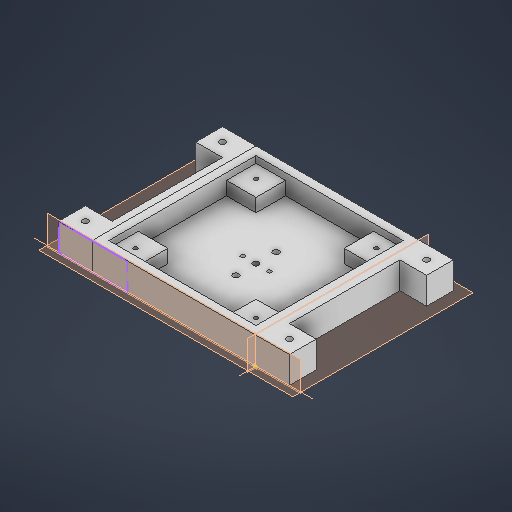
# Autodesk Inventor part: Unterteil
Saved by Autodesk Inventor 2026.2 (Build 302298000, 298)
## iProperties
Created: 2026-04-09
Part Number: Unterteil
Material: Generisch
Document SubType Name: Modeling
Designer: linda
Density: 1 g/cm^3
Appearance: Vorgabe
Author: linda
Autodesk Inventor part; units mm, degrees
sketch "Skizze1" plane through (0, 0, 0) normal (0, 1, 0) x (-1, 0, 0)
  line L0 (0, 0) -> (122.5, 0)
  line L1 (122.5, 0) -> (122.5, -122.5)
  line L2 (122.5, -122.5) -> (0, -122.5)
  line L3 (0, -122.5) -> (0, 0)
  dimension "d0" = 122.5
  dimension "d1" = 122.5
  constraints: 8 end point, 2 parallel, 1 horizontal, 1 perpendicular
  measures "d0" distance of L1.end L2.end
  measures "d1" distance of L0.end L1.end
extrude "Extrusion1" add sketch "Skizze1" along normal blind 20
sketch "Skizze2" plane through (0, 20, 0) normal (0, 1, 0) x (1, 0, 0)
  line L0 (-6.25042, 6.249757) -> (-116.25042, 6.249757)
  line L1 (-116.25042, 6.249757) -> (-116.25042, 116.249757)
  line L2 (-116.25042, 116.249757) -> (-6.25042, 116.249757)
  line L3 (-6.25042, 116.249757) -> (-6.25042, 6.249757)
  point P0 (0, 0)
  dimension "d6" = 110
  dimension "d7" = 110
  constraints: 8 end point, 2 parallel, 1 horizontal, 1 perpendicular
  measures "d6" distance of L1.end L2.end
  measures "d7" distance of L0.end L1.end
extrude "Extrusion2" cut sketch "Skizze2" against normal blind 15
sketch "Skizze3" plane through (0, 5, 0) normal (0, 1, 0) x (1, 0, 0)
  line L0 (-6.250425, 6.249784) -> (-21.250425, 6.249784)
  line L1 (-21.250425, 6.249784) -> (-21.250425, 21.249784)
  line L2 (-21.250425, 21.249784) -> (-6.250425, 21.249784)
  line L3 (-6.250425, 21.249784) -> (-6.250425, 6.249784)
  line L4 (-6.250425, 116.250797) -> (-21.250425, 116.250797)
  line L5 (-21.250425, 116.250797) -> (-21.250425, 101.250797)
  line L6 (-21.250425, 101.250797) -> (-6.250425, 101.250797)
  line L7 (-6.250425, 101.250797) -> (-6.250425, 116.250797)
  line L8 (-116.250374, 116.249733) -> (-101.250374, 116.249733)
  line L9 (-101.250374, 116.249733) -> (-101.250374, 101.249733)
  line L10 (-101.250374, 101.249733) -> (-116.250374, 101.249733)
  line L11 (-116.250374, 101.249733) -> (-116.250374, 116.249733)
  line L12 (-116.250374, 6.249784) -> (-101.250374, 6.249784)
  line L13 (-101.250374, 6.249784) -> (-101.250374, 21.249784)
  line L14 (-101.250374, 21.249784) -> (-116.250374, 21.249784)
  line L15 (-116.250374, 21.249784) -> (-116.250374, 6.249784)
  point P0 (0, 0)
  dimension "d10" = 15
  dimension "d11" = 15
  dimension "d12" = 15
  dimension "d13" = 15
  dimension "d14" = 15
  dimension "d15" = 15
  dimension "d16" = 15
  dimension "d17" = 15
  constraints: 32 end point, 8 parallel, 4 horizontal, 4 perpendicular, 1 point on line
  measures "d10" distance of L1.end L2.end
  measures "d11" distance of L0.end L1.end
  measures "d12" distance of L6.end L5.end
  measures "d13" distance of L5.end L4.end
  measures "d14" distance of L9.end L10.end
  measures "d15" distance of L8.end L9.end
  measures "d16" distance of L14.end L13.end
  measures "d17" distance of L13.end L12.end
extrude "Extrusion3" add sketch "Skizze3" along normal blind 10
sketch "Skizze4" plane through (0, 5, 0) normal (0, 1, 0) x (1, 0, 0)
  line L0 (-21.249763, 21.249862) -> (-28.320831, 28.32093)
  line L1 (-21.249763, 21.249862) -> (-11.249763, 21.249862) construction
  line L2 (-28.320831, 28.32093) -> (-6.25074, 28.32093)
  line L3 (-6.25074, 28.32093) -> (-6.25074, 6.250839)
  line L4 (-6.25074, 6.250839) -> (-28.320831, 6.250839)
  line L5 (-28.320831, 6.250839) -> (-28.320831, 28.32093)
  line L6 (-21.250382, 101.250909) -> (-28.32145, 94.179842)
  line L7 (-21.250382, 101.250909) -> (-11.250382, 101.250909) construction
  line L8 (-6.250411, 116.249742) -> (-28.32145, 116.249742)
  line L9 (-28.32145, 116.249742) -> (-28.32145, 94.179842)
  line L10 (-28.32145, 94.179842) -> (-6.250411, 94.179842)
  line L11 (-6.250411, 94.179842) -> (-6.250411, 116.249742)
  line L12 (-101.251429, 21.249862) -> (-94.180362, 28.32093)
  line L13 (-101.251429, 21.249862) -> (-91.251429, 21.249862) construction
  line L14 (-94.180362, 28.32093) -> (-116.250453, 28.32093)
  line L15 (-116.250453, 28.32093) -> (-116.250453, 6.250839)
  line L16 (-116.250453, 6.250839) -> (-94.180362, 6.250839)
  line L17 (-94.180362, 6.250839) -> (-94.180362, 28.32093)
  line L18 (-101.251429, 101.250909) -> (-94.180362, 94.179842)
  line L19 (-101.251429, 101.250909) -> (-91.251429, 101.250909) construction
  line L20 (-94.180362, 94.179842) -> (-116.250453, 94.179842)
  line L21 (-116.250453, 94.179842) -> (-116.250453, 116.249933)
  line L22 (-116.250453, 116.249933) -> (-94.180362, 116.249933)
  line L23 (-94.180362, 116.249933) -> (-94.180362, 94.179842)
  point P0 (0, 0)
  dimension "d20" = 10
  dimension "d21" = 135
  dimension "d22" = 10
  dimension "d23" = 135
  dimension "d24" = 10
  dimension "d25" = 45
  dimension "d26" = 10
  dimension "d27" = 45
  constraints: 48 end point, 8 horizontal, 8 parallel, 4 equal length, 4 perpendicular, 2 point on line
  measures "d20" distance of L0.start L0.end
  measures "d21" angle of L1 L0
  measures "d22" distance of L6.start L6.end
  measures "d23" angle of L6 L7
  measures "d24" distance of L12.start L12.end
  measures "d25" angle of L13 L12
  measures "d26" distance of L18.start L18.end
  measures "d27" angle of L18 L19
extrude "Extrusion4" add sketch "Skizze4" along normal blind 10
sketch "Skizze5" plane through (0, 15, 0) normal (0, 1, 0) x (1, 0, 0)
  line L0 (-28.320831, 28.32093) -> (-28.320831, 6.250839)
  line L1 (-6.25074, 28.32093) -> (-28.320831, 28.32093)
  point P0 (0, 0)
  point P1 (-16.250831, 16.25093)
  dimension "d30" = 12.07
  dimension "d31" = 12.07
  measures "d30" distance from line of L0 point (-16.251, 16.251)
  measures "d31" distance from line of L1 point (-16.251, 16.251)
hole "Bohrung1" at (-16.250831, 15, -16.25093) direction (0, -1, 0) diameter 3 end through all
sketch "Skizze6" plane through (0, 15, 0) normal (0, 1, 0) x (1, 0, 0)
  line L0 (-94.180362, 6.250839) -> (-94.180362, 28.32093)
  line L1 (-94.180362, 28.32093) -> (-116.25042, 28.32093)
  point P0 (0, 0)
  point P1 (-106.250362, 16.25093)
  dimension "d39" = 12.07
  dimension "d40" = 12.07
  measures "d39" distance from line of L0 point (-106.25, 16.251)
  measures "d40" distance from line of L1 point (-106.25, 16.251)
hole "Bohrung2" at (-106.250362, 15, -16.25093) direction (0, -1, 0) diameter 3 end through all
sketch "Skizze7" plane through (0, 15, 0) normal (0, 1, 0) x (1, 0, 0)
  line L0 (-28.32145, 94.179842) -> (-6.25042, 94.179842)
  line L1 (-28.32145, 116.249742) -> (-28.32145, 94.179842)
  point P0 (0, 0)
  point P1 (-16.25145, 106.249842)
  dimension "d48" = 12.07
  dimension "d49" = 12.07
  measures "d48" distance from line of L0 point (-16.251, 106.25)
  measures "d49" distance from line of L1 point (-16.251, 106.25)
hole "Bohrung3" at (-16.25145, 15, -106.249842) direction (0, -1, 0) diameter 3 end through all
sketch "Skizze8" plane through (0, 15, 0) normal (0, 1, 0) x (1, 0, 0)
  line L0 (-116.25042, 94.179842) -> (-94.180362, 94.179842)
  line L1 (-94.180362, 94.179842) -> (-94.180362, 116.249757)
  point P0 (0, 0)
  point P1 (-106.250362, 106.249842)
  dimension "d57" = 12.07
  dimension "d58" = 12.07
  measures "d57" distance from line of L0 point (-106.25, 106.25)
  measures "d58" distance from line of L1 point (-106.25, 106.25)
hole "Bohrung4" at (-106.250362, 15, -106.249842) direction (0, -1, 0) diameter 3 end through all
thread "Gewinde1" size "M3x0.5" class "6H" standard "ANSI Metric M Profile" full length
thread "Gewinde2" size "M3x0.5" class "6H" standard "ANSI Metric M Profile" full length
thread "Gewinde3" size "M3x0.5" class "6H" standard "ANSI Metric M Profile" full length
thread "Gewinde4" size "M3x0.5" class "6H" standard "ANSI Metric M Profile" full length
sketch "Skizze9" plane through (0, 5, 0) normal (0, 1, 0) x (1, 0, 0)
  line L0 (0, 122.5) -> (-122.5, 122.5) projected
  line L1 (0, 0) -> (0, 122.5) projected
  point P0 (-61.25, 61.25)
  dimension "d74" = 61.25
  dimension "d75" = 61.25
  measures "d74" distance from line of L0 point (-61.25, 61.25)
  measures "d75" distance from line of L1 point (-61.25, 61.25)
hole "Bohrung5" at (-61.25, 5, -61.25) direction (0, -1, 0) diameter 4.4 end through all
thread "Gewinde5" size "M5x0.8" class "6H" standard "ANSI Metric M Profile" full length
sketch "Skizze10" plane through (0, 5, 0) normal (0, 1, 0) x (1, 0, 0)
  circle A0 centre (-61.25, 61.25) radius 2.2
  line L0 (-94.180362, 116.249757) -> (-94.180362, 94.179842)
  line L1 (-94.180362, 94.179842) -> (-116.25042, 94.179842)
  line L2 (-116.25042, 28.32093) -> (-116.25042, 94.179842)
  line L3 (-116.25042, 28.32093) -> (-94.180362, 28.32093)
  line L4 (-94.180362, 28.32093) -> (-94.180362, 6.250839)
  line L5 (-94.180362, 6.250839) -> (-101.250374, 6.250839)
  line L6 (-101.250374, 6.250839) -> (-101.250374, 6.249784)
  line L7 (-101.250374, 6.249784) -> (-116.250374, 6.249784)
  line L8 (-116.250374, 6.249784) -> (-116.250374, 6.250839)
  line L9 (-116.250374, 6.250839) -> (-116.25042, 6.250839)
  line L10 (-116.25042, 6.249757) -> (-116.25042, 6.250839)
  line L11 (-6.25042, 6.249757) -> (-116.25042, 6.249757)
  line L12 (-6.250425, 6.249784) -> (-6.25042, 6.249757)
  line L13 (-6.250425, 6.249784) -> (-21.250425, 6.249784)
  line L14 (-21.250425, 6.249784) -> (-21.250425, 6.250839)
  line L15 (-21.250425, 6.250839) -> (-28.320831, 6.250839)
  line L16 (-28.320831, 6.250839) -> (-28.320831, 28.32093)
  line L17 (-28.320831, 28.32093) -> (-6.25074, 28.32093)
  line L18 (-6.25074, 28.32093) -> (-6.25074, 21.249784)
  line L19 (-6.25074, 21.249784) -> (-6.250425, 21.249784)
  line L20 (-6.250411, 94.179842) -> (-6.250425, 21.249784)
  line L21 (-6.250411, 94.179842) -> (-28.32145, 94.179842)
  line L22 (-28.32145, 94.179842) -> (-28.32145, 116.249742)
  line L23 (-28.32145, 116.249742) -> (-21.250425, 116.249742)
  line L24 (-21.250425, 116.249742) -> (-21.250425, 116.249757)
  line L25 (-94.180362, 116.249757) -> (-21.250425, 116.249757)
  line L26 (-61.25, 61.25) -> (-71.25, 61.25)
  line L27 (-61.25, 61.25) -> (-51.25, 61.25)
  point P0 (0, 0)
  dimension "d85" = 10
  dimension "d86" = 10
  constraints: 4 end point, 2 horizontal
  measures "d85" distance of L26.start L26.end
  measures "d86" distance of L26.start L27.end
hole "Bohrung6" at (-71.25, 5, -61.25) direction (0, -1, 0) diameter 3 end through all
sketch "Skizze11" plane through (0, 5, 0) normal (0, 1, 0) x (1, 0, 0)
  circle A0 centre (-61.25, 61.25) radius 2.2
  line L0 (-61.25, 61.25) -> (-52.345425, 61.25)
  line L1 (-61.25, 61.25) -> (-51.25, 61.25)
  point P0 (0, 0)
  dimension "d94" = 10
  constraints: 4 end point, 1 horizontal, 1 point on line
  measures "d94" distance of L0.start L1.end
hole "Bohrung7" at (-51.25, 5, -61.25) direction (0, -1, 0) diameter 3 end through all
sketch "Skizze12" plane through (0, 5, 0) normal (0, 1, 0) x (1, 0, 0)
  circle A0 centre (-61.25, 61.25) radius 2.2 projected
  line L0 (-61.25, 61.25) -> (-61.25, 76.25)
  point P0 (0, 0)
  dimension "d102" = 15
  constraints: 2 end point, 1 vertical
  measures "d102" distance of L0.start L0.end
hole "Bohrung8" at (-61.25, 5, -76.25) direction (0, -1, 0) diameter 4.5 end through all
sketch "Skizze13" plane through (0, 5, 0) normal (0, 1, 0) x (1, 0, 0)
  circle A0 centre (-61.25, 61.25) radius 2.2 projected
  line L0 (-61.25, 61.25) -> (-61.25, 46.25)
  point P0 (0, 0)
  dimension "d110" = 15
  constraints: 2 end point, 1 vertical
  measures "d110" distance of L0.start L0.end
hole "Bohrung9" at (-61.25, 5, -46.25) direction (0, -1, 0) diameter 4.5 end through all
sketch "Skizze14" plane through (0, 20, 0) normal (0, 1, 0) x (1, 0, 0)
  line L0 (0, 0) -> (5, 0)
  line L1 (5, 0) -> (5, 122.5)
  line L2 (5, 122.5) -> (0, 122.5)
  line L3 (0, 122.5) -> (0, 0)
  line L4 (-122.500054, 0) -> (-127.500054, 0)
  line L5 (-127.500054, 0) -> (-127.500054, 122.5)
  line L6 (-127.500054, 122.5) -> (-122.500054, 122.5)
  line L7 (-122.500054, 122.5) -> (-122.500054, 0)
  dimension "d118" = 5
  dimension "d119" = 122.5
  dimension "d120" = 5
  dimension "d121" = 122.5
  constraints: 16 end point, 4 parallel, 2 horizontal, 2 perpendicular
  measures "d118" distance of L2.end L1.end
  measures "d119" distance of L1.end L0.end
  measures "d120" distance of L5.end L6.end
  measures "d121" distance of L4.end L5.end
extrude "Extrusion5" add sketch "Skizze14" against normal blind 20
sketch "Skizze17" plane through (5, 20, 0) normal (1, 0, 0) x (0, 0, -1)
  line L0 (0, -20) -> (20, -20)
  line L1 (20, -20) -> (20, 0)
  line L2 (20, 0) -> (0, 0)
  line L3 (0, 0) -> (0, -20)
  line L4 (122.499971, 0) -> (102.499971, 0)
  line L5 (102.499971, 0) -> (102.499971, -20)
  line L6 (102.499971, -20) -> (122.499971, -20)
  line L7 (122.499971, -20) -> (122.499971, 0)
  dimension "d135" = 20
  dimension "d136" = 20
  dimension "d137" = 20
  dimension "d138" = 20
  constraints: 16 end point, 4 parallel, 2 horizontal, 2 perpendicular, 1 point on line
  measures "d135" distance of L2.end L1.end
  measures "d136" distance of L1.end L0.end
  measures "d137" distance of L6.end L5.end
  measures "d138" distance of L5.end L4.end
extrude "Extrusion6" add sketch "Skizze17" along normal blind 20
sketch "Skizze18" plane through (-127.500054, 20, -122.5) normal (-1, 0, 0) x (0, 0, 1)
  line L0 (122.5, -20) -> (102.5, -20)
  line L1 (102.5, -20) -> (102.5, 0)
  line L2 (102.5, 0) -> (122.5, 0)
  line L3 (122.5, 0) -> (122.5, -20)
  line L4 (-0.000021, 0) -> (19.999979, 0)
  line L5 (19.999979, 0) -> (19.999979, -20)
  line L6 (19.999979, -20) -> (-0.000021, -20)
  line L7 (-0.000021, -20) -> (-0.000021, 0)
  dimension "d141" = 20
  dimension "d142" = 20
  dimension "d143" = 20
  dimension "d144" = 20
  constraints: 16 end point, 4 parallel, 2 horizontal, 2 perpendicular, 1 point on line
  measures "d141" distance of L1.end L2.end
  measures "d142" distance of L0.end L1.end
  measures "d143" distance of L5.end L6.end
  measures "d144" distance of L4.end L5.end
extrude "Extrusion7" add sketch "Skizze18" along normal blind 20
sketch "Skizze20" plane through (0, 20, 0) normal (0, 1, 0) x (1, 0, 0)
  line L0 (5, 122.499971) -> (25, 122.499971)
  line L1 (25, 122.499971) -> (25, 102.499971)
  line L2 (-122.5, 0) -> (25, 0)
  line L3 (25, 20) -> (25, 0)
  point P0 (0, 0)
  point P1 (15, 112.499971)
  point P2 (15, 10)
  dimension "d147" = 10
  dimension "d148" = 10
  dimension "d149" = 10
  dimension "d150" = 10
  measures "d147" distance from line of L0 point (15, 112.5)
  measures "d148" distance from line of L1 point (15, 112.5)
  measures "d149" distance from line of L2 point (15, 10)
  measures "d150" distance from line of L3 point (15, 10)
hole "Bohrung11" at (15, 20, -112.499971) at (15, 20, -10) direction (0, -1, 0) diameter 4.5 end through all
sketch "Skizze21" plane through (0, 20, 0) normal (0, 1, 0) x (1, 0, 0)
  line L0 (-127.500054, 20) -> (-147.500054, 20)
  line L1 (-147.500054, 0) -> (-147.500054, 20)
  line L2 (-127.500054, 122.500021) -> (-147.500054, 122.500021)
  line L3 (-147.500054, 102.500021) -> (-147.500054, 122.500021)
  point P0 (0, 0)
  point P1 (-137.500054, 10)
  point P2 (-137.500054, 112.500021)
  dimension "d158" = 10
  dimension "d159" = 10
  dimension "d160" = 10
  dimension "d161" = 10
  measures "d158" distance from line of L0 point (-137.5, 10)
  measures "d159" distance from line of L1 point (-137.5, 10)
  measures "d160" distance from line of L2 point (-137.5, 112.5)
  measures "d161" distance from line of L3 point (-137.5, 112.5)
hole "Bohrung12" at (-137.500054, 20, -10) at (-137.500054, 20, -112.500021) direction (0, -1, 0) diameter 4.5 end through all
sketch "Skizze22" plane through (-122.5, 0, 0) normal (0, 0, 1) x (1, 0, 0)
  line L0 (-24.949836, 0) -> (26.477746, 0)
  line L1 (26.477746, 0) -> (26.477746, 19.853841)
  line L2 (26.477746, 19.853841) -> (-24.949836, 19.853841)
  line L3 (-24.949836, 19.853841) -> (-24.949836, 0)
  point P0 (122.5, 0)
  constraints: 8 end point, 2 parallel, 1 horizontal, 1 perpendicular
